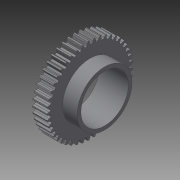
# Autodesk Inventor part: M-0.5 Zb-4mm M-0.7 Zb-5mm mN 21104500
Saved by Autodesk Inventor 2017.3 (Build 213256000, 256)
## iProperties
Category: PARTsolutions
Company: MAEDLER
Created: 2018-08-16
Part Number: M-0.5 Zb-4mm M-0.7 Zb-5mm mN 21104500
Material: Generic
Catalog Web Link: www.cadenas.de
Description: M-0.5 Zb-4mm M-0.7 Zb-5mm mN-Spur Gears, Steel, Module 0.5 and 0,7
Vendor: MAEDLER
Document SubType Name: Modeling
Designer: psadmin
Manufacturer: MAEDLER
Mass: 16 g
Surface Area: 15.9637 cm^2
Volume: 2.1259 cm^3
Density: 1 g/cm^3
Appearance: PSOLRGB-175-175-175
PSOL_IDENT_0: {$CADENAS_DATA\23d-libs\maedler\antriebselemente\stirnzahnraeder\stirnzahnraeder_stahl\modul_0.5_und
PSOL_IDENT_1: _0.7\m-0.5_zb-4mm_m-0.7_zb-5mm_mn.prj},237 {VTYP=3D},{NB=M-0.5 Zb-4mm M-0.7 Zb-5mm mN 21104500},{LIN
PSOL_IDENT_2: A=M-0.5 Zb-4mm M-0.7 Zb-5mm mN 21104500},{NN=M-0.5 Zb-4mm M-0.7 Zb-5mm mN},{DATE=27.10.2015 07:21:56
PSOL_IDENT_3: },{GEOMDATE=11.05.2009 09:51:00},{VERSION=},{LINEID=260},{WBVAR=},{WBNUMERIC=}  {NB=M-0.5 Zb-4mm M-0
PSOL_IDENT_4: .7 Zb-5mm mN 21104500},{LINA=M-0.5 Zb-4mm M-0.7 Zb-5mm mN 21104500},{KT=DUMMY},{ARTNR=21104500},{WST=
PSOL_IDENT_5: 11SMnPb30},{M=0.5},{Z=45},{PDF=PDF Katalogseite},{B1=4.0},{DA=23.50},{D=22.50},{NL=4},{ND=15},{B=5},
PSOL_IDENT_6: {MD=13.4},{GEW=16.000}
NN: M-0.5 Zb-4mm M-0.7 Zb-5mm mN
NT: Spur Gears, Steel, Module 0.5 and 0,7
NB: M-0.5 Zb-4mm M-0.7 Zb-5mm mN 21104500
NBSYN: M-0.5 Zb-4mm M-0.7 Zb-5mm mN $ARTNR.
LINA: M-0.5 Zb-4mm M-0.7 Zb-5mm mN 21104500
ARTNR: 21104500
WST: 11SMnPb30
M: 0.5
Z: 45
PDF: PDF Katalogseite
B1: 4
DA: 23.5
D: 22.5
NL: 4
ND: 15
B: 5
MD: 13.4
GEW: 16
SUPPLIER: MAEDLER
ARTICLENO: M-0.5 Zb-4mm M-0.7 Zb-5mm mN 21104500
BOMINFO: M-0.5 Zb-4mm M-0.7 Zb-5mm mN 21104500
CREATOR: CADENAS GmbH
Title: M-0.5 Zb-4mm M-0.7 Zb-5mm mN 21104500
Author: Cadenas PARTsolutions
Comments: Spur Gears, Steel, Module 0.5 and 0,7
Autodesk Inventor part; units mm, degrees
ref_plane "YZ Plane" through (0, 0, 0) normal (1, 0, 0) x (0, 1, 0)
ref_plane "XZ Plane" through (0, 0, 0) normal (0, 1, 0) x (-1, 0, 0)
ref_plane "XY Plane" through (0, 0, 0) normal (0, 0, 1) x (1, 0, 0)
sketch "Skizze_1" plane through (0, 0, 0) normal (1, 0, 0) x (0, 1, 0)
  arc A0 (-0.2435, 11.7475) -> (-0.5766, 11.7358) centre (0, 0) ccw
  line L0 (-0.5766, 11.7358) -> (-0.7473, 11.2252)
  line L1 (-0.7473, 11.2252) -> (-0.8746, 10.7144)
  arc A1 (-0.8746, 10.7144) -> (-1.3721, 10.6621) centre (0, 0) ccw
  line L2 (-1.3721, 10.6621) -> (-1.6029, 11.1352)
  line L3 (-1.6029, 11.1352) -> (-1.876, 11.5993)
  arc A2 (-1.876, 11.5993) -> (-2.2043, 11.5414) centre (0, 0) ccw
  line L4 (-2.2043, 11.5414) -> (-2.3022, 11.0119)
  line L5 (-2.3022, 11.0119) -> (-2.3572, 10.4884)
  arc A3 (-2.3572, 10.4884) -> (-2.8427, 10.3673) centre (0, 0) ccw
  line L6 (-2.8427, 10.3673) -> (-3.137, 10.8038)
  line L7 (-3.137, 10.8038) -> (-3.4721, 11.2253)
  arc A4 (-3.4721, 11.2253) -> (-3.7891, 11.1223) centre (0, 0) ccw
  line L8 (-3.7891, 11.1223) -> (-3.8124, 10.5843)
  line L9 (-3.8124, 10.5843) -> (-3.794, 10.0582)
  arc A5 (-3.794, 10.0582) -> (-4.2579, 9.8708) centre (0, 0) ccw
  line L10 (-4.2579, 9.8708) -> (-4.6101, 10.262)
  line L11 (-4.6101, 10.262) -> (-5.0005, 10.6328)
  arc A6 (-5.0005, 10.6328) -> (-5.3001, 10.4867) centre (0, 0) ccw
  line L12 (-5.3001, 10.4867) -> (-5.2483, 9.9508)
  line L13 (-5.2483, 9.9508) -> (-5.1569, 9.4323)
  arc A7 (-5.1569, 9.4323) -> (-5.5902, 9.1822) centre (0, 0) ccw
  line L14 (-5.5902, 9.1822) -> (-5.9934, 9.5206)
  line L15 (-5.9934, 9.5206) -> (-6.4317, 9.8334)
  arc A8 (-6.4317, 9.8334) -> (-6.708, 9.647) centre (0, 0) ccw
  line L16 (-6.708, 9.647) -> (-6.5821, 9.1235)
  line L17 (-6.5821, 9.1235) -> (-6.4195, 8.6228)
  arc A9 (-6.4195, 8.6228) -> (-6.8137, 8.3148) centre (0, 0) ccw
  line L18 (-6.8137, 8.3148) -> (-7.2601, 8.5938)
  line L19 (-7.2601, 8.5938) -> (-7.7376, 8.8426)
  arc A10 (-7.7376, 8.8426) -> (-7.9854, 8.6196) centre (0, 0) ccw
  line L20 (-7.9854, 8.6196) -> (-7.7878, 8.1186)
  line L21 (-7.7878, 8.1186) -> (-7.557, 7.6455)
  arc A11 (-7.557, 7.6455) -> (-7.9046, 7.2856) centre (0, 0) ccw
  line L22 (-7.9046, 7.2856) -> (-8.3855, 7.4997)
  line L23 (-8.3855, 7.4997) -> (-8.893, 7.6797)
  arc A12 (-8.893, 7.6797) -> (-9.1072, 7.4243) centre (0, 0) ccw
  line L24 (-9.1072, 7.4243) -> (-8.8419, 6.9558)
  line L25 (-8.8419, 6.9558) -> (-8.5475, 6.5193)
  arc A13 (-8.5475, 6.5193) -> (-8.8416, 6.1146) centre (0, 0) ccw
  line L26 (-8.8416, 6.1146) -> (-9.3476, 6.2597)
  line L27 (-9.3476, 6.2597) -> (-9.8752, 6.3673)
  arc A14 (-9.8752, 6.3673) -> (-10.0519, 6.0846) centre (0, 0) ccw
  line L28 (-10.0519, 6.0846) -> (-9.7239, 5.6575)
  line L29 (-9.7239, 5.6575) -> (-9.3717, 5.2663)
  arc A15 (-9.3717, 5.2663) -> (-9.6066, 4.8246) centre (0, 0) ccw
  line L30 (-9.6066, 4.8246) -> (-10.1279, 4.8979)
  line L31 (-10.1279, 4.8979) -> (-10.6653, 4.9309)
  arc A16 (-10.6653, 4.9309) -> (-10.8009, 4.6264) centre (0, 0) ccw
  line L32 (-10.8009, 4.6264) -> (-10.4167, 4.2492)
  line L33 (-10.4167, 4.2492) -> (-10.0134, 3.9108)
  arc A17 (-10.0134, 3.9108) -> (-10.1845, 3.4407) centre (0, 0) ccw
  line L34 (-10.1845, 3.4407) -> (-10.7109, 3.4407)
  line L35 (-10.7109, 3.4407) -> (-11.2477, 3.3986)
  arc A18 (-11.2477, 3.3986) -> (-11.3396, 3.0782) centre (0, 0) ccw
  line L36 (-11.3396, 3.0782) -> (-10.9067, 2.7581)
  line L37 (-10.9067, 2.7581) -> (-10.4602, 2.4791)
  arc A19 (-10.4602, 2.4791) -> (-10.5642, 1.9898) centre (0, 0) ccw
  line L38 (-10.5642, 1.9898) -> (-11.0856, 1.9165)
  line L39 (-11.0856, 1.9165) -> (-11.6113, 1.8002)
  arc A20 (-11.6113, 1.8002) -> (-11.6577, 1.4701) centre (0, 0) ccw
  line L40 (-11.6577, 1.4701) -> (-11.1844, 1.2133)
  line L41 (-11.1844, 1.2133) -> (-10.7035, 0.9992)
  arc A21 (-10.7035, 0.9992) -> (-10.7384, 0.5001) centre (0, 0) ccw
  line L42 (-10.7384, 0.5001) -> (-11.2444, 0.355)
  line L43 (-11.2444, 0.355) -> (-11.7488, 0.1667)
  arc A22 (-11.7488, 0.1667) -> (-11.7488, -0.1667) centre (0, 0) ccw
  line L44 (-11.7488, -0.1667) -> (-11.2444, -0.355)
  line L45 (-11.2444, -0.355) -> (-10.7384, -0.5001)
  arc A23 (-10.7384, -0.5001) -> (-10.7035, -0.9992) centre (0, 0) ccw
  line L46 (-10.7035, -0.9992) -> (-11.1844, -1.2133)
  line L47 (-11.1844, -1.2133) -> (-11.6577, -1.4701)
  arc A24 (-11.6577, -1.4701) -> (-11.6113, -1.8002) centre (0, 0) ccw
  line L48 (-11.6113, -1.8002) -> (-11.0856, -1.9165)
  line L49 (-11.0856, -1.9165) -> (-10.5642, -1.9898)
  arc A25 (-10.5642, -1.9898) -> (-10.4602, -2.4791) centre (0, 0) ccw
  line L50 (-10.4602, -2.4791) -> (-10.9067, -2.7581)
  line L51 (-10.9067, -2.7581) -> (-11.3396, -3.0782)
  arc A26 (-11.3396, -3.0782) -> (-11.2477, -3.3986) centre (0, 0) ccw
  line L52 (-11.2477, -3.3986) -> (-10.7109, -3.4407)
  line L53 (-10.7109, -3.4407) -> (-10.1845, -3.4407)
  arc A27 (-10.1845, -3.4407) -> (-10.0134, -3.9108) centre (0, 0) ccw
  line L54 (-10.0134, -3.9108) -> (-10.4167, -4.2492)
  line L55 (-10.4167, -4.2492) -> (-10.8009, -4.6264)
  arc A28 (-10.8009, -4.6264) -> (-10.6653, -4.9309) centre (0, 0) ccw
  line L56 (-10.6653, -4.9309) -> (-10.1279, -4.8979)
  line L57 (-10.1279, -4.8979) -> (-9.6066, -4.8246)
  arc A29 (-9.6066, -4.8246) -> (-9.3717, -5.2663) centre (0, 0) ccw
  line L58 (-9.3717, -5.2663) -> (-9.7239, -5.6575)
  line L59 (-9.7239, -5.6575) -> (-10.0519, -6.0846)
  arc A30 (-10.0519, -6.0846) -> (-9.8752, -6.3673) centre (0, 0) ccw
  line L60 (-9.8752, -6.3673) -> (-9.3476, -6.2597)
  line L61 (-9.3476, -6.2597) -> (-8.8416, -6.1146)
  arc A31 (-8.8416, -6.1146) -> (-8.5475, -6.5193) centre (0, 0) ccw
  line L62 (-8.5475, -6.5193) -> (-8.8419, -6.9558)
  line L63 (-8.8419, -6.9558) -> (-9.1072, -7.4243)
  arc A32 (-9.1072, -7.4243) -> (-8.893, -7.6797) centre (0, 0) ccw
  line L64 (-8.893, -7.6797) -> (-8.3855, -7.4997)
  line L65 (-8.3855, -7.4997) -> (-7.9046, -7.2856)
  arc A33 (-7.9046, -7.2856) -> (-7.557, -7.6455) centre (0, 0) ccw
  line L66 (-7.557, -7.6455) -> (-7.7878, -8.1186)
  line L67 (-7.7878, -8.1186) -> (-7.9854, -8.6196)
  arc A34 (-7.9854, -8.6196) -> (-7.7376, -8.8426) centre (0, 0) ccw
  line L68 (-7.7376, -8.8426) -> (-7.2601, -8.5938)
  line L69 (-7.2601, -8.5938) -> (-6.8137, -8.3148)
  arc A35 (-6.8137, -8.3148) -> (-6.4195, -8.6228) centre (0, 0) ccw
  line L70 (-6.4195, -8.6228) -> (-6.5821, -9.1235)
  line L71 (-6.5821, -9.1235) -> (-6.708, -9.647)
  arc A36 (-6.708, -9.647) -> (-6.4317, -9.8334) centre (0, 0) ccw
  line L72 (-6.4317, -9.8334) -> (-5.9934, -9.5206)
  line L73 (-5.9934, -9.5206) -> (-5.5902, -9.1822)
  arc A37 (-5.5902, -9.1822) -> (-5.1569, -9.4323) centre (0, 0) ccw
  line L74 (-5.1569, -9.4323) -> (-5.2483, -9.9508)
  line L75 (-5.2483, -9.9508) -> (-5.3001, -10.4867)
  arc A38 (-5.3001, -10.4867) -> (-5.0005, -10.6328) centre (0, 0) ccw
  line L76 (-5.0005, -10.6328) -> (-4.6101, -10.262)
  line L77 (-4.6101, -10.262) -> (-4.2579, -9.8708)
  arc A39 (-4.2579, -9.8708) -> (-3.794, -10.0582) centre (0, 0) ccw
  line L78 (-3.794, -10.0582) -> (-3.8124, -10.5843)
  line L79 (-3.8124, -10.5843) -> (-3.7891, -11.1223)
  arc A40 (-3.7891, -11.1223) -> (-3.4721, -11.2253) centre (0, 0) ccw
  line L80 (-3.4721, -11.2253) -> (-3.137, -10.8038)
  line L81 (-3.137, -10.8038) -> (-2.8427, -10.3673)
  arc A41 (-2.8427, -10.3673) -> (-2.3572, -10.4884) centre (0, 0) ccw
  line L82 (-2.3572, -10.4884) -> (-2.3022, -11.0119)
  line L83 (-2.3022, -11.0119) -> (-2.2043, -11.5414)
  arc A42 (-2.2043, -11.5414) -> (-1.876, -11.5993) centre (0, 0) ccw
  line L84 (-1.876, -11.5993) -> (-1.6029, -11.1352)
  line L85 (-1.6029, -11.1352) -> (-1.3721, -10.6621)
  arc A43 (-1.3721, -10.6621) -> (-0.8746, -10.7144) centre (0, 0) ccw
  line L86 (-0.8746, -10.7144) -> (-0.7473, -11.2252)
  line L87 (-0.7473, -11.2252) -> (-0.5766, -11.7358)
  arc A44 (-0.5766, -11.7358) -> (-0.2435, -11.7475) centre (0, 0) ccw
  line L88 (-0.2435, -11.7475) -> (-0.0376, -11.2499)
  line L89 (-0.0376, -11.2499) -> (0.1251, -10.7493)
  arc A45 (0.1251, -10.7493) -> (0.6251, -10.7318) centre (0, 0) ccw
  line L90 (0.6251, -10.7318) -> (0.8223, -11.2199)
  line L91 (0.8223, -11.2199) -> (1.0623, -11.7019)
  arc A46 (1.0623, -11.7019) -> (1.3938, -11.667) centre (0, 0) ccw
  line L92 (1.3938, -11.667) -> (1.5285, -11.1457)
  line L93 (1.5285, -11.1457) -> (1.6199, -10.6273)
  arc A47 (1.6199, -10.6273) -> (2.1126, -10.5404) centre (0, 0) ccw
  line L94 (2.1126, -10.5404) -> (2.3758, -10.9963)
  line L95 (2.3758, -10.9963) -> (2.6806, -11.4401)
  arc A48 (2.6806, -11.4401) -> (3.004, -11.3595) centre (0, 0) ccw
  line L96 (3.004, -11.3595) -> (3.0648, -10.8245)
  line L97 (3.0648, -10.8245) -> (3.0831, -10.2984)
  arc A49 (3.0831, -10.2984) -> (3.5589, -10.1438) centre (0, 0) ccw
  line L98 (3.5589, -10.1438) -> (3.883, -10.5586)
  line L99 (3.883, -10.5586) -> (4.2467, -10.9557)
  arc A50 (4.2467, -10.9557) -> (4.5557, -10.8309) centre (0, 0) ccw
  line L100 (4.5557, -10.8309) -> (4.5414, -10.2926)
  line L101 (4.5414, -10.2926) -> (4.4864, -9.7691)
  arc A51 (4.4864, -9.7691) -> (4.936, -9.5498) centre (0, 0) ccw
  line L102 (4.936, -9.5498) -> (5.3147, -9.9155)
  line L103 (5.3147, -9.9155) -> (5.7301, -10.2581)
  arc A52 (5.7301, -10.2581) -> (6.0187, -10.0914) centre (0, 0) ccw
  line L104 (6.0187, -10.0914) -> (5.9297, -9.5604)
  line L105 (5.9297, -9.5604) -> (5.8023, -9.0496)
  arc A53 (5.8023, -9.0496) -> (6.2171, -8.7699) centre (0, 0) ccw
  line L106 (6.2171, -8.7699) -> (6.643, -9.0793)
  line L107 (6.643, -9.0793) -> (7.102, -9.3608)
  arc A54 (7.102, -9.3608) -> (7.3646, -9.1556) centre (0, 0) ccw
  line L108 (7.3646, -9.1556) -> (7.2025, -8.6421)
  line L109 (7.2025, -8.6421) -> (7.0053, -8.154)
  arc A55 (7.0053, -8.154) -> (7.3771, -7.8193) centre (0, 0) ccw
  line L110 (7.3771, -7.8193) -> (7.8419, -8.0664)
  line L111 (7.8419, -8.0664) -> (8.3356, -8.2813)
  arc A56 (8.3356, -8.2813) -> (8.5672, -8.0415) centre (0, 0) ccw
  line L112 (8.5672, -8.0415) -> (8.3352, -7.5556)
  line L113 (8.3352, -7.5556) -> (8.072, -7.0997)
  arc A57 (8.072, -7.0997) -> (8.3935, -6.7165) centre (0, 0) ccw
  line L114 (8.3935, -6.7165) -> (8.8882, -6.8965)
  line L115 (8.8882, -6.8965) -> (9.407, -7.0406)
  arc A58 (9.407, -7.0406) -> (9.603, -6.7709) centre (0, 0) ccw
  line L116 (9.603, -6.7709) -> (9.3056, -6.3221)
  line L117 (9.3056, -6.3221) -> (8.9815, -5.9072)
  arc A59 (8.9815, -5.9072) -> (9.2466, -5.483) centre (0, 0) ccw
  line L118 (9.2466, -5.483) -> (9.7615, -5.5924)
  line L119 (9.7615, -5.5924) -> (10.2953, -5.6629)
  arc A60 (10.2953, -5.6629) -> (10.4518, -5.3686) centre (0, 0) ccw
  line L120 (10.4518, -5.3686) -> (10.0949, -4.9654)
  line L121 (10.0949, -4.9654) -> (9.7162, -4.5998)
  arc A61 (9.7162, -4.5998) -> (9.9197, -4.1427) centre (0, 0) ccw
  line L122 (9.9197, -4.1427) -> (10.4448, -4.1794)
  line L123 (10.4448, -4.1794) -> (10.9833, -4.1749)
  arc A62 (10.9833, -4.1749) -> (11.0973, -3.8617) centre (0, 0) ccw
  line L124 (11.0973, -3.8617) -> (10.6877, -3.5122)
  line L125 (10.6877, -3.5122) -> (10.2618, -3.2028)
  arc A63 (10.2618, -3.2028) -> (10.3997, -2.7218) centre (0, 0) ccw
  line L126 (10.3997, -2.7218) -> (10.9249, -2.6851)
  line L127 (10.9249, -2.6851) -> (11.4574, -2.6057)
  arc A64 (11.4574, -2.6057) -> (11.5267, -2.2797) centre (0, 0) ccw
  line L128 (11.5267, -2.2797) -> (11.0725, -1.9906)
  line L129 (11.0725, -1.9906) -> (10.6077, -1.7434)
  arc A65 (10.6077, -1.7434) -> (10.6773, -1.248) centre (0, 0) ccw
  line L130 (10.6773, -1.248) -> (11.1922, -1.1385)
  line L131 (11.1922, -1.1385) -> (11.7086, -0.9858)
  arc A66 (11.7086, -0.9858) -> (11.7318, -0.6533) centre (0, 0) ccw
  line L132 (11.7318, -0.6533) -> (11.2418, -0.4302)
  line L133 (11.2418, -0.4302) -> (10.7471, -0.2501)
  arc A67 (10.7471, -0.2501) -> (10.7471, 0.2501) centre (0, 0) ccw
  line L134 (10.7471, 0.2501) -> (11.2418, 0.4302)
  line L135 (11.2418, 0.4302) -> (11.7318, 0.6533)
  arc A68 (11.7318, 0.6533) -> (11.7086, 0.9858) centre (0, 0) ccw
  line L136 (11.7086, 0.9858) -> (11.1922, 1.1385)
  line L137 (11.1922, 1.1385) -> (10.6773, 1.248)
  arc A69 (10.6773, 1.248) -> (10.6077, 1.7434) centre (0, 0) ccw
  line L138 (10.6077, 1.7434) -> (11.0725, 1.9906)
  line L139 (11.0725, 1.9906) -> (11.5267, 2.2797)
  arc A70 (11.5267, 2.2797) -> (11.4574, 2.6057) centre (0, 0) ccw
  line L140 (11.4574, 2.6057) -> (10.9249, 2.6851)
  line L141 (10.9249, 2.6851) -> (10.3997, 2.7218)
  arc A71 (10.3997, 2.7218) -> (10.2618, 3.2028) centre (0, 0) ccw
  line L142 (10.2618, 3.2028) -> (10.6877, 3.5122)
  line L143 (10.6877, 3.5122) -> (11.0973, 3.8617)
  arc A72 (11.0973, 3.8617) -> (10.9833, 4.1749) centre (0, 0) ccw
  line L144 (10.9833, 4.1749) -> (10.4448, 4.1794)
  line L145 (10.4448, 4.1794) -> (9.9197, 4.1427)
  arc A73 (9.9197, 4.1427) -> (9.7162, 4.5998) centre (0, 0) ccw
  line L146 (9.7162, 4.5998) -> (10.0949, 4.9654)
  line L147 (10.0949, 4.9654) -> (10.4518, 5.3686)
  arc A74 (10.4518, 5.3686) -> (10.2953, 5.6629) centre (0, 0) ccw
  line L148 (10.2953, 5.6629) -> (9.7615, 5.5924)
  line L149 (9.7615, 5.5924) -> (9.2466, 5.483)
  arc A75 (9.2466, 5.483) -> (8.9815, 5.9072) centre (0, 0) ccw
  line L150 (8.9815, 5.9072) -> (9.3056, 6.3221)
  line L151 (9.3056, 6.3221) -> (9.603, 6.7709)
  arc A76 (9.603, 6.7709) -> (9.407, 7.0406) centre (0, 0) ccw
  line L152 (9.407, 7.0406) -> (8.8882, 6.8965)
  line L153 (8.8882, 6.8965) -> (8.3935, 6.7165)
  arc A77 (8.3935, 6.7165) -> (8.072, 7.0997) centre (0, 0) ccw
  line L154 (8.072, 7.0997) -> (8.3352, 7.5556)
  line L155 (8.3352, 7.5556) -> (8.5672, 8.0415)
  arc A78 (8.5672, 8.0415) -> (8.3356, 8.2813) centre (0, 0) ccw
  line L156 (8.3356, 8.2813) -> (7.8419, 8.0664)
  line L157 (7.8419, 8.0664) -> (7.3771, 7.8193)
  arc A79 (7.3771, 7.8193) -> (7.0053, 8.154) centre (0, 0) ccw
  line L158 (7.0053, 8.154) -> (7.2025, 8.6421)
  line L159 (7.2025, 8.6421) -> (7.3646, 9.1556)
  arc A80 (7.3646, 9.1556) -> (7.102, 9.3608) centre (0, 0) ccw
  line L160 (7.102, 9.3608) -> (6.643, 9.0793)
  line L161 (6.643, 9.0793) -> (6.2171, 8.7699)
  arc A81 (6.2171, 8.7699) -> (5.8023, 9.0496) centre (0, 0) ccw
  line L162 (5.8023, 9.0496) -> (5.9297, 9.5604)
  line L163 (5.9297, 9.5604) -> (6.0187, 10.0914)
  arc A82 (6.0187, 10.0914) -> (5.7301, 10.2581) centre (0, 0) ccw
  line L164 (5.7301, 10.2581) -> (5.3147, 9.9155)
  line L165 (5.3147, 9.9155) -> (4.936, 9.5498)
  arc A83 (4.936, 9.5498) -> (4.4864, 9.7691) centre (0, 0) ccw
  line L166 (4.4864, 9.7691) -> (4.5414, 10.2926)
  line L167 (4.5414, 10.2926) -> (4.5557, 10.8309)
  arc A84 (4.5557, 10.8309) -> (4.2467, 10.9557) centre (0, 0) ccw
  line L168 (4.2467, 10.9557) -> (3.883, 10.5586)
  line L169 (3.883, 10.5586) -> (3.5589, 10.1438)
  arc A85 (3.5589, 10.1438) -> (3.0831, 10.2984) centre (0, 0) ccw
  line L170 (3.0831, 10.2984) -> (3.0648, 10.8245)
  line L171 (3.0648, 10.8245) -> (3.004, 11.3595)
  arc A86 (3.004, 11.3595) -> (2.6806, 11.4401) centre (0, 0) ccw
  line L172 (2.6806, 11.4401) -> (2.3758, 10.9963)
  line L173 (2.3758, 10.9963) -> (2.1126, 10.5404)
  arc A87 (2.1126, 10.5404) -> (1.6199, 10.6273) centre (0, 0) ccw
  line L174 (1.6199, 10.6273) -> (1.5285, 11.1457)
  line L175 (1.5285, 11.1457) -> (1.3938, 11.667)
  arc A88 (1.3938, 11.667) -> (1.0623, 11.7019) centre (0, 0) ccw
  line L176 (1.0623, 11.7019) -> (0.8223, 11.2199)
  line L177 (0.8223, 11.2199) -> (0.6251, 10.7318)
  arc A89 (0.6251, 10.7318) -> (0.1251, 10.7493) centre (0, 0) ccw
  line L178 (0.1251, 10.7493) -> (-0.0376, 11.2499)
  line L179 (-0.0376, 11.2499) -> (-0.2435, 11.7475)
  constraints: 360 end point, 180 point on circle, 90 centre point
extrude "Extrusion1" add sketch "Skizze_1" along normal mid plane 4
sketch "Skizze_2" plane through (0, 0, 0) normal (0, 0, 1) x (1, 0, 0)
  line L0 (6, 0) -> (2, 0)
  line L1 (2, 0) -> (2, 7.5)
  line L2 (2, 7.5) -> (6, 7.5)
  line L3 (6, 7.5) -> (6, 0)
  line L4 (6, 0) -> (2, 0)
  constraints: 10 end point
revolve "Revolution1" add sketch "Skizze_2" angle 360 about axis through (6, 0, 0) along (1, 0, 0)
sketch "Skizze_3" plane through (6, 0, 0) normal (1, 0, 0) x (0, 1, 0)
  circle A0 centre (0, 0) radius 2.5
  constraints: 1 centre point
extrude "Extrusion2" cut sketch "Skizze_3" along normal mid plane 16
sketch "Skizze4" plane through (-2, 0, 0) normal (-1, 0, 0) x (0, 0, 1)
  circle A0 centre (0, 0) radius 2.5 projected
  circle A1 centre (0, 0) radius 6.5
  dimension "d5" = 13
  constraints: 1 centre point, 1 coincident
  measures "d5" diameter of A1
extrude "Extrusion3" cut sketch "Skizze4" against normal through all
body "Solid1"
